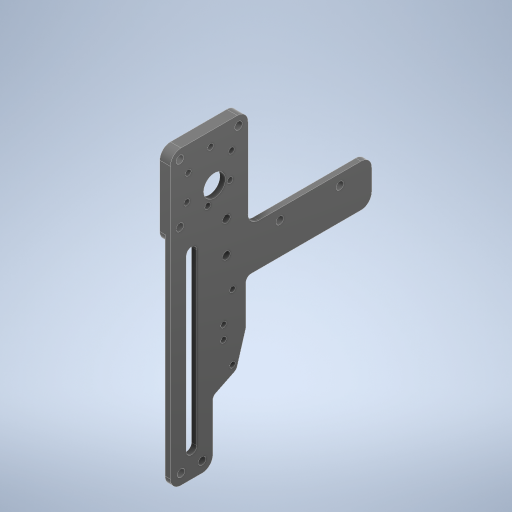
# Autodesk Inventor part: Side Plate 2.0-bck
Saved by Autodesk Inventor 2024 (Build 280153000, 153)
## iProperties
Created: 2024-01-10
Part Number: Side Plate 2.0-bck
Material: Generic
Document SubType Name: Modeling
Designer: Greg
Density: 1 g/cm^3
Appearance: Smooth - Black
Author: Greg
## iProperties of the stored document MemberDocs/xYzscaup5Hshz0zq1Inerlj2pKf
Created: 2024-01-10
Part Number: Side Plate 2.0-bck
Material: Generic
Document SubType Name: Modeling
Designer: Greg
Density: 1 g/cm^3
Appearance: Smooth - Black
Author: Greg
Autodesk Inventor part; units mm, degrees
note: some values were not read from the file. Chosen so that the rebuilt part matches the saved one: edges of "Fillet1"; direction of "Hole2"; direction of "Hole3".
ref_plane "YZ Plane" through (0, 0, 0) normal (1, 0, 0) x (0, 1, 0)
ref_plane "XZ Plane" through (0, 0, 0) normal (0, 1, 0) x (-1, 0, 0)
ref_plane "XY Plane" through (0, 0, 0) normal (0, 0, 1) x (1, 0, 0)
sketch "Sketch1" plane through (0, 0, 0) normal (1, 0, 0) x (0, 1, 0)
  line L0 (0, 0) -> (127, 0)
  line L1 (127, 0) -> (127, -25.4)
  line L2 (127, -25.4) -> (0, -25.4)
  line L3 (0, -25.4) -> (0, 0)
  line L4 (127, -25.4) -> (36.4241, -25.4)
  line L5 (15.875, -12.7) -> (117.475, -12.7) construction
  line L6 (15.875, -15.875) -> (117.475, -15.875)
  line L7 (117.475, -9.525) -> (15.875, -9.525)
  arc A0 (15.875, -9.525) -> (15.875, -15.875) centre (15.875, -12.7) ccw
  arc A1 (117.475, -15.875) -> (117.475, -9.525) centre (117.475, -12.7) ccw
  line L8 (6.35, -6.35) -> (6.35, -19.05) construction
  point P0 (66.675, -12.7)
  point P1 (127, -12.7)
  point P2 (6.35, -12.7)
  point P3 (0, -12.7)
  point P4 (12.7, -12.7)
  point P5 (120.65, -12.7)
  dimension "d0" = 6.35
  dimension "d1" = 101.6
  dimension "d2" = 9.525
  dimension "d3" = 6.35
  dimension "d4" = 12.7
  dimension "d5" = 6.35
  dimension "d6" = 6.35
  constraints: 20 end point, 6 point on circle, 4 midpoint, 4 tangent, 3 horizontal, 3 parallel, 2 centre point, 2 horizontal alignment, 1 perpendicular, 1 vertical, 1 vertical alignment
  measures "d0" diameter of A1
  measures "d1" distance of L5.start L5.end
  measures "d2" distance between parallel lines of L0 L7
  measures "d3" distance between parallel lines of L3 L8
  measures "d4" distance of L8.start L8.end
  measures "d5" distance from line of point (12.7, -12.7) L8
  measures "d6" distance from line of point (120.65, -12.7) L1
extrude "Extrusion1" add sketch "Sketch1" along normal blind 3.175
sketch "Sketch2" plane through (3.175, 0, 0) normal (1, 0, 0) x (0, 0, -1)
  line L0 (25.4, 0) -> (25.4, 127) projected
  line L1 (25.4, 88.9) -> (120.65, 88.9)
  line L2 (120.65, 88.9) -> (120.65, 114.3)
  line L3 (120.65, 114.3) -> (25.4, 114.3)
  line L4 (25.4, 114.3) -> (25.4, 88.9)
  line L5 (0, 0) -> (25.4, 0) projected
  point P0 (25.4, 114.3)
  dimension "d9" = 88.9
  dimension "d10" = 95.25
  dimension "d11" = 25.4
  constraints: 8 end point, 2 parallel, 1 horizontal, 1 perpendicular, 1 point on line
  measures "d9" distance between parallel lines of L5 L1
  measures "d10" distance between parallel lines of L2 L0
  measures "d11" distance of L1.end L2.end
extrude "Extrusion2" add sketch "Sketch2" against normal up to surface (3.175 mm away)
sketch "Sketch3" plane through (3.175, 0, 0) normal (1, 0, 0) x (0, 0, -1)
  circle A0 centre (23.2625, 151.85) radius 18.5 construction
  line L0 (0, 127) -> (0, 0) projected
  arc A1 (15.875, 117.475) -> (9.525, 117.475) centre (12.7, 117.475) ccw projected
  line L1 (12.7, 117.475) -> (12.7, 19.05) construction
  arc A2 (9.525, 15.875) -> (15.875, 15.875) centre (12.7, 15.875) ccw projected
  line L2 (0, 127) -> (0, 175.1125)
  line L3 (0, 175.1125) -> (46.525, 175.1125)
  line L4 (46.525, 175.1125) -> (46.525, 114.3)
  line L5 (25.4, 114.3) -> (120.65, 114.3) projected
  line L6 (25.4, 0) -> (25.4, 88.9) projected
  circle A3 centre (26.416, 145.6006) radius 6.5
  line L7 (25.4, 127) -> (0, 127) projected
  line L8 (25.4, 114.3) -> (25.4, 127) projected
  circle A4 centre (23.2625, 151.85) radius 7
  circle A5 centre (26.416, 145.6006) radius 10.541 construction
  line L9 (15.875, 117.475) -> (15.875, 15.875) projected
  circle A6 centre (23.2625, 151.85) radius 0.25
  point P0 (12.7, 120.65)
  point P1 (23.2625, 175.1125)
  dimension "d95" = 14
  dimension "d14" = 37
  dimension "d20" = 4.7625
  dimension "d21" = 13
  dimension "d96" = 21.082
  dimension "d97" = 4.7625
  dimension "d98" = 6.35
  dimension "d99" = 0.5
  constraints: 8 end point, 4 centre point, 3 coincident, 2 perpendicular, 2 point on circle, 2 vertical, 1 midpoint, 1 point on line, 1 tangent, 1 vertical alignment, 3 other
  measures "d14" diameter of A0
  measures "d20" distance edge to line of A0 L3
  measures "d21" diameter of A3
  measures "d96" diameter of A5
  measures "d97" distance edge to line of A0 L2
  measures "d98" distance edge to line of A0 L7
  measures "d99" diameter of A6
extrude "Extrusion3" add sketch "Sketch3" against normal up to surface (3.175 mm away) contours L2 L3 L4 L5 L8 L7 | A3 A4 picked at (24.876, 154.206)
sketch "Sketch4" plane through (0, 0, 0) normal (-1, 0, 0) x (0, 0, 1)
  line L0 (0, 0) -> (-25.4, 0) projected
  line L1 (-20.6375, 12.7) -> (-20.6375, 125.4125)
  line L2 (-20.6375, 125.4125) -> (0, 125.4125)
  line L3 (0, 175.1125) -> (0, 0) projected
  line L4 (-120.65, 114.3) -> (-120.65, 88.9) projected
  line L5 (-120.65, 95.25) -> (-46.525, 95.25)
  line L6 (-46.525, 114.3) -> (-46.525, 175.1125) projected
  line L7 (-46.525, 95.25) -> (-46.525, 114.3)
  line L8 (-120.65, 88.9) -> (-25.4, 88.9) projected
  line L9 (-15.875, 117.475) -> (-15.875, 15.875) projected
  line L10 (0, 175.1125) -> (-46.525, 175.1125) projected
  arc A0 (-9.525, 117.475) -> (-15.875, 117.475) centre (-12.7, 117.475) ccw projected
  line L11 (-25.4, 0) -> (-25.4, 88.9) projected
  circle A1 centre (-26.416, 145.6006) radius 6.5 projected
  line L12 (-20.6375, 12.7) -> (-25.4, 12.7)
  circle A2 centre (-23.2625, 151.85) radius 0.25 projected
  point P0 (-23.1933, 146.0566)
  point P1 (-23.1093, 146.0184)
  dimension "d24" = 6.35
  dimension "d25" = 4.7625
  dimension "d26" = 4.7625
  dimension "d29" = 12.7
  constraints: 10 end point, 3 perpendicular, 3 point on line, 1 horizontal, 1 vertical, 2 other
  measures "d24" distance between parallel lines of L8 L5
  measures "d25" distance between parallel lines of L9 L1
  measures "d26" distance edge to line of A0 L2
  measures "d29" distance between parallel lines of L0 L12
extrude "Extrusion4" add sketch "Sketch4" along normal blind 3.175 contours L2 L1 L12 L11 L8 L4 L5 L7 L6 L10 L3 | A1 | A2
sketch "Sketch19" plane through (3.175, 0, 0) normal (1, 0, 0) x (0, 0, -1)
  circle A0 centre (23.2625, 151.85) radius 0.25 projected
  circle A1 centre (26.416, 145.6006) radius 6.5 projected
  line L0 (23.2625, 151.85) -> (26.416, 145.6006) construction
  line L1 (23.2625, 151.85) -> (36.6541, 158.6075) construction
  point P0 (0, 0)
  point P1 (23.1933, 146.0566)
  point P2 (23.1093, 146.0184)
  dimension "d100" = 15
  constraints: 4 end point, 1 coincident, 1 perpendicular, 2 other
  measures "d100" distance of L0.start L1.end
hole "Hole4" at (3.175, 158.6075, -36.6541) direction (-1, 0, 0) diameter 3.4036 end through all clearance for "Flat Head Machine Screw" size "M3" standard "Ansi Metric M Profile"
pattern_circular "Circular Pattern2" count 6 over 360 about axis through (3.175, 151.85, -23.2625) along (-1, 0, 0) of "Hole4"
sketch "Sketch14" plane through (-3.175, 0, 0) normal (-1, 0, 0) x (0, 0, 1)
  circle A0 centre (-23.2625, 151.85) radius 18.5
  circle A1 centre (-23.2625, 151.85) radius 0.25 projected
  point P0 (0, 0)
  dimension "d75" = 37
  constraints: 1 centre point, 1 coincident
  measures "d75" diameter of A0
extrude "Extrusion10" cut sketch "Sketch14" against normal up to surface (3.175 mm away) contours A0 | A1
sketch "Sketch10" plane through (-3.175, 0, 0) normal (-1, 0, 0) x (0, 0, 1)
  line L0 (-46.525, 95.25) -> (-46.525, 114.3) projected
  line L1 (-25.4, 88.9) -> (-120.65, 88.9) projected
  line L2 (-46.525, 95.25) -> (-120.65, 95.25)
  line L3 (-120.65, 95.25) -> (-120.65, 88.9)
  line L4 (-120.65, 88.9) -> (-46.525, 88.9)
  line L5 (-46.525, 88.9) -> (-46.525, 95.25)
  point P0 (0, 0)
  point P1 (-46.525, 88.9)
  constraints: 8 end point, 2 parallel, 1 horizontal, 1 perpendicular
extrude "Extrusion9" add sketch "Sketch10" along normal blind 25.4
fillet "Fillet1" radius 6.35 11 edges at (-12.7, 88.9, -120.65) (1.5875, 114.3, -120.65) (1.5875, 114.3, -46.525) (0, 88.9, -25.4) (1.5875, 0, -25.4) (1.5875, 0, 0) (-1.5875, 125.4125, -20.6375) (0, 175.1125, 0) (0, 175.1125, -46.525) (-1.5875, 125.4125, 0) (-1.5875, 95.25, -46.525)
fillet "Fillet2" radius 2.3813 2 edges at (-1.5875, 12.7, -25.4) (-1.5875, 12.7, -20.6375)
fillet "Fillet3" radius 19.05 1 edges at (-3.175, 92.075, -46.525)
sketch "Sketch12" plane through (-3.175, 0, 0) normal (-1, 0, 0) x (0, 0, 1)
  line L0 (-19.05, 6.35) -> (-6.35, 6.35) construction
  line L1 (-6.35, 0) -> (-19.05, 0) projected
  line L2 (-40.8562, 134.2563) -> (-5.6688, 134.2563) construction
  line L3 (-5.6688, 134.2563) -> (-5.6688, 169.4437) construction
  line L4 (-5.6688, 169.4437) -> (-40.8562, 169.4437) construction
  line L5 (-40.8562, 169.4437) -> (-40.8562, 134.2563) construction
  line L6 (-40.8562, 134.2563) -> (-5.6688, 169.4437) construction
  line L7 (-5.6688, 134.2563) -> (-40.8562, 169.4437) construction
  arc A0 (0, 168.7625) -> (-6.35, 175.1125) centre (-6.35, 168.7625) ccw projected
  line L8 (-46.525, 168.7625) -> (-46.525, 101.6) projected
  line L9 (-46.525, 124.7313) -> (-20.6375, 124.7313) construction
  line L10 (-20.6375, 119.0625) -> (-20.6375, 15.0813) projected
  line L11 (-120.65, 107.95) -> (-120.65, 95.25) projected
  circle A1 centre (-40.8562, 169.4437) radius 4 construction
  circle A2 centre (-23.2625, 151.85) radius 0.25 projected
  circle A3 centre (-23.2625, 151.85) radius 18.5 projected
  point P0 (0, 0)
  point P1 (-12.7, 6.35)
  point P2 (-12.7, 0)
  point P3 (-33.5812, 124.7313)
  point P4 (-33.5812, 105.6813)
  point P5 (-101.6, 107.95)
  point P6 (-65.575, 107.95)
  point P7 (-23.1093, 146.0184)
  point P8 (-23.1933, 146.0566)
  point P9 (-31.9832, 168.1656)
  point P10 (-14.5418, 168.1656)
  dimension "d60" = 6.35
  dimension "d61" = 12.7
  dimension "d64" = 9.525
  dimension "d65" = 19.05
  dimension "d66" = 19.05
  dimension "d67" = 19.05
  dimension "d92" = 8
  dimension "d111" = 2.3813
  constraints: 16 end point, 7 coincident, 4 midpoint, 3 horizontal, 2 horizontal alignment, 2 parallel, 2 perpendicular, 2 point on line, 2 vertical alignment, 1 centre point, 1 other
  measures "d60" distance between parallel lines of L1 L0
  measures "d61" distance of L0.start L0.end
  measures "d64" distance between parallel lines of L2 L9
  measures "d65" distance of point (-33.581, 105.681) point (-33.581, 124.731)
  measures "d66" distance from line of L11 point (-101.6, 107.95)
  measures "d67" distance from line of L8 point (-65.575, 107.95)
  measures "d92" diameter of A1
hole "Hole2" at (-3.175, 107.95, -101.6) at (-3.175, 105.6813, -33.5812) at (-3.175, 124.7313, -33.5812) at (-3.175, 107.95, -65.575) at (-3.175, 169.4437, -40.8562) at (-3.175, 169.4437, -5.6688) at (-3.175, 134.2563, -5.6688) at (-3.175, 6.35, -6.35) at (-3.175, 6.35, -19.05) direction (1, 0, 0) diameter 4.4958 depth 6.35 clearance for "Flat Head Machine Screw (82)" size "#8" standard "Ansi Unified Screw Threads"
sketch "Sketch15" plane through (0, 95.25, -52.875) normal (0, 1, 0) x (1, 0, 0)
  line L0 (28.575, -0.4477) -> (28.575, 74.9206) construction
  line L1 (3.175, 61.425) -> (3.175, 0) projected
  line L2 (-7.425, 55.05) -> (-7.425, 43.05) construction
  line L3 (-7.425, 43.05) -> (-7.425, 31.05) construction
  line L4 (-7.425, 31.05) -> (-7.425, 19.05) construction
  line L5 (-22.225, -6.35) -> (-28.575, -6.35) projected
  point P0 (0, -52.875)
  dimension "d79" = 50.8
  dimension "d80" = 72
  dimension "d81" = 12
  dimension "d82" = 25.4
  constraints: 8 end point, 4 collinear, 2 vertical
  measures "d79" diameter of L1 L0
  measures "d80" diameter of L2.start L0
  measures "d81" distance of L2.start L2.end
  measures "d82" distance from line of L5 L4.end
hole "Hole3" at (-7.425, 95.25, -107.925) at (-7.425, 95.25, -95.925) at (-7.425, 95.25, -83.925) at (-7.425, 95.25, -71.925) direction (0, -1, 0) diameter 3.2766 depth 6.35 clearance for "Flat Head Machine Screw (82)" size "#4" standard "Ansi Unified Screw Threads"
sketch "Sketch16" plane through (0, 95.25, -52.875) normal (0, 1, 0) x (1, 0, 0)
  line L0 (-28.575, -6.35) -> (-28.575, 67.775) projected
  line L1 (-28.575, 67.775) -> (-14.85, 67.775)
  line L2 (-14.85, 67.775) -> (-14.85, -7.8355)
  line L3 (-14.85, -7.8355) -> (-28.575, -7.8355)
  line L4 (-28.575, -7.8355) -> (-28.575, 67.775)
  line L5 (0, 67.775) -> (-28.575, 67.775) projected
  line L6 (-14.85, 67.775) -> (0, 67.775)
  circle A0 centre (-7.425, 55.05) radius 1.6383 projected
  arc A1 (-3.175, -25.4) -> (-22.225, -6.35) centre (-22.225, -25.4) ccw projected
  point P0 (0, -52.875)
  point P1 (-7.425, 67.775)
  constraints: 10 end point, 2 horizontal, 2 parallel, 1 midpoint, 1 perpendicular, 1 point on circle, 1 vertical alignment
extrude "Extrusion11" cut sketch "Sketch16" against normal blind 25.4 contours L0 L1 L2 L3 L4
sketch "Sketch20" plane through (3.175, 0, 0) normal (1, 0, 0) x (0, 0, -1)
  circle A0 centre (23.2625, 151.85) radius 0.25 projected
  point P0 (0, 0)
extrude "Extrusion13" add sketch "Sketch20" against normal up to surface (3.175 mm away)
sketch "Sketch17" plane through (0, 151.85, -23.2625) normal (-1, 0, 0) x (0, 0, 1)
  circle A0 centre (-3.1535, -6.2494) radius 6.5 projected
  circle A1 centre (0, 0) radius 18.5 projected
  point P0 (23.2625, -151.85)
extrude "Extrusion12" [suppressed]
sketch "Sketch21" plane through (3.175, 0, 0) normal (1, 0, 0) x (0, 0, -1)
  line L0 (27.4462, 49.1158) -> (31.877, 70.665) construction
  line L1 (31.877, 70.665) -> (41.6721, 68.651) construction
  line L2 (41.6721, 68.651) -> (37.2413, 47.1018) construction
  line L3 (37.2413, 47.1018) -> (27.4462, 49.1158) construction
  line L4 (23.9035, 46.7814) -> (29.5427, 74.2077)
  line L5 (29.5427, 74.2077) -> (45.2148, 70.9853)
  line L6 (45.2148, 70.9853) -> (39.5756, 43.559)
  line L7 (39.5756, 43.559) -> (23.9035, 46.7814)
  line L8 (25.4, 6.35) -> (25.4, 82.55) projected
  line L9 (22.924, 46.9828) -> (15.875, 12.7) construction
  line L10 (22.924, 46.9828) -> (23.9035, 46.7814) construction
  arc A0 (9.525, 15.875) -> (15.875, 15.875) centre (12.7, 15.875) ccw projected
  line L11 (37.2413, 86.2482) -> (41.6721, 64.699) construction
  line L12 (41.6721, 64.699) -> (31.877, 62.685) construction
  line L13 (31.877, 62.685) -> (27.4462, 84.2342) construction
  line L14 (27.4462, 84.2342) -> (37.2413, 86.2482) construction
  line L15 (39.5756, 89.791) -> (45.2148, 62.3647)
  line L16 (45.2148, 62.3647) -> (29.5427, 59.1423)
  line L17 (29.5427, 59.1423) -> (23.9035, 86.5686)
  line L18 (23.9035, 86.5686) -> (39.5756, 89.791)
  line L19 (22.924, 86.3672) -> (15.875, 120.65) construction
  arc A1 (15.875, 117.475) -> (9.525, 117.475) centre (12.7, 117.475) ccw projected
  line L20 (22.924, 86.3672) -> (23.9035, 86.5686) construction
  line L21 (45.2148, 62.3647) -> (45.2148, 88.9)
  line L22 (31.75, 88.9) -> (114.3, 88.9) projected
  line L23 (45.2148, 62.3647) -> (39.5756, 43.559)
  line L24 (39.5756, 43.559) -> (25.4, 36.6202)
  arc A2 (31.75, 88.9) -> (25.4, 82.55) centre (31.75, 82.55) ccw projected
  point P0 (0, 0)
  point P1 (31.7396, 45.1702)
  point P2 (26.7231, 60.4946)
  point P3 (12.7, 12.7)
  point P4 (31.7396, 88.1798)
  point P5 (42.3952, 76.0778)
  point P6 (12.7, 120.65)
  point P7 (25.4, 46.4737)
  point P8 (43.3641, 61.9842)
  point P9 (39.7588, 88.9)
  point P10 (27.9939, 66.675)
  point P11 (43.3641, 71.3658)
  point P12 (25.4, 54.0597)
  point P13 (25.4, 79.2903)
  point P14 (44.3286, 66.675)
  point P15 (27.5585, 87.3201)
  point P16 (25.9656, 85.1697)
  point P17 (45.2148, 70.9853)
  point P18 (45.2148, 70.9853)
  point P19 (35.2424, 88.9)
  dimension "d3" = 6.35
  dimension "d114" = 22
  dimension "d115" = 10
  dimension "d117" = 28
  dimension "d118" = 3
  dimension "d119" = 3
  dimension "d121" = 35
  dimension "d122" = 1
  dimension "d123" = 6.477
  dimension "d128" = 22
  dimension "d129" = 10
  dimension "d130" = 16
  dimension "d131" = 28
  dimension "d132" = 3
  dimension "d133" = 3
  dimension "d134" = 35
  dimension "d137" = 1
  dimension "d140" = 37.7
  dimension "d149" = 3
  constraints: 46 end point, 8 parallel, 8 perpendicular, 6 coincident, 4 midpoint, 3 vertical alignment, 2 horizontal alignment, 2 point on circle, 2 point on line, 1 vertical
  measures "d114" distance of L1.end L2.end
  measures "d115" distance of L0.end L1.end
  measures "d117" distance of L5.end L6.end
  measures "d118" distance between parallel lines of L0 L4
  measures "d119" distance between parallel lines of L5 L1
  measures "d121" distance of L9.start L9.end
  measures "d122" distance between parallel lines of L4 L9
  measures "d123" distance from line of L8 point (31.877, 70.665)
  measures "d128" distance of L13.start L13.end
  measures "d129" distance of L11.end L13.start
  measures "d130" distance of L15.end L17.start
  measures "d131" distance of L17.start L17.end
  measures "d132" distance between parallel lines of L11 L15
  measures "d133" distance between parallel lines of L16 L12
  measures "d134" distance of L19.start L19.end
  measures "d137" distance of L19.start L17.end
  measures "d140" angle of L7 L24
  measures "d149" distance between parallel lines of L6 L2
extrude "Extrusion14" add sketch "Sketch21" against normal up to surface (3.175 mm away)
hole "Hole5" at (3.175, 70.665, -31.877) at (3.175, 47.1018, -37.2413) at (3.175, 86.2482, -37.2413) at (3.175, 62.685, -31.877) direction (-1, 0, 0) diameter 3.2766 end through all clearance for "Flat Head Machine Screw (82)" size "#4" standard "Ansi Unified Screw Threads"
fillet "Fillet5" radius 3.175 4 edges at (1.5875, 36.6202, -25.4) (1.5875, 43.559, -39.5756) (1.5875, 62.3647, -45.2148) (1.5875, 88.9, -45.2148)
equation "\"d6\" = d5"
equation "\"d66\" = d65"
body "Solid1"
